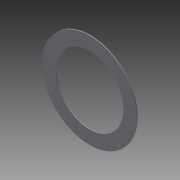
# Autodesk Inventor part: back layer of front
Saved by Autodesk Inventor 2013 (Build 170138000, 138)
## iProperties
Created: 2013-07-18
Part Number: back layer of front
Material: Generic
Document SubType Name: Modeling
Designer: owner
Density: 1 g/cm^3
Author: owner
Autodesk Inventor part; units mm, degrees
ref_plane "YZ Plane" through (0, 0, 0) normal (1, 0, 0) x (0, 1, 0)
ref_plane "XZ Plane" through (0, 0, 0) normal (0, 1, 0) x (-1, 0, 0)
ref_plane "XY Plane" through (0, 0, 0) normal (0, 0, 1) x (1, 0, 0)
sketch "Sketch1" plane through (0, 0, 0) normal (0, 0, 1) x (1, 0, 0)
  circle A0 centre (0, 0) radius 355.6
  circle A1 centre (0, 0) radius 254
  circle A2 centre (0, -330.2) radius 3.175
  circle A3 centre (119.282, -307.9023) radius 3.175
  circle A4 centre (222.4543, -244.0207) radius 3.175
  circle A5 centre (295.5829, -147.1828) radius 3.175
  circle A6 centre (328.7914, -30.467) radius 3.175
  circle A7 centre (317.5948, 90.3635) radius 3.175
  circle A8 centre (263.5053, 198.99) radius 3.175
  circle A9 centre (173.8279, 280.7417) radius 3.175
  circle A10 centre (60.6741, 324.5777) radius 3.175
  circle A11 centre (-60.6741, 324.5777) radius 3.175
  circle A12 centre (-173.8279, 280.7417) radius 3.175
  circle A13 centre (-263.5053, 198.99) radius 3.175
  circle A14 centre (-317.5948, 90.3635) radius 3.175
  circle A15 centre (-328.7914, -30.467) radius 3.175
  circle A16 centre (-295.5829, -147.1828) radius 3.175
  circle A17 centre (-222.4543, -244.0207) radius 3.175
  circle A18 centre (-119.282, -307.9023) radius 3.175
  dimension "d0" = 711.2
  dimension "d1" = 508
  dimension "d3" = 6.35
  dimension "d6" = 360
  constraints: 19 centre point, 2 coincident, 35 other
  measures "d0" diameter of A0
  measures "d1" diameter of A1
  measures "d3" diameter of A2
extrude "Extrusion1" add sketch "Sketch1" along normal blind 6.35
body "Solid1"
